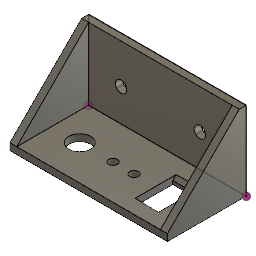
Switch Bracket v2 (Autodesk Fusion 360 design; units mm, degrees)
Autodesk Fusion 360 part; units mm, degrees
note: some values were not read from the file. Set by a fixed rule: which sketch regions a step uses.
sketch "Sketch1" plane through (0, 0, 0) normal (0, 1, 0) x (1, 0, 0)
  line L0 (45, 22.5) -> (-45, 22.5)
  line L1 (-45, 22.5) -> (-45, -22.5)
  line L2 (-45, -22.5) -> (45, -22.5)
  line L3 (45, -22.5) -> (45, 22.5)
  line L4 (45, 22.5) -> (-45, -22.5) construction
  line L5 (-45, 22.5) -> (45, -22.5) construction
  dimension "d1" = 45
  dimension "d2" = 90
  constraint perpendicular L0 L1
  constraint parallel L0 L2
  constraint parallel L1 L3
  constraint horizontal L0
  constraint coincident L4 origin
  constraint coincident L5 origin
  measures "d1" distance of L0.start L2.end L0.end
  measures "d2" distance of L0.start L0.end
extrude "Extrude1" add sketch "Sketch1" along normal blind 4
sketch "Sketch2" plane through (0, 0, -22.5) normal (0, 0, -1) x (-1, 0, 0)
  line L0 (45, 0) -> (-45, 0)
  line L1 (-45, 0) -> (-45, 45)
  line L2 (-45, 45) -> (45, 45)
  line L3 (45, 45) -> (45, 0)
  point P0 (-45, 0)
  point P1 (45, 0)
  dimension "d12" = 45
  constraint horizontal L0
  constraint vertical L1
  constraint horizontal L2
  constraint vertical L3
  constraint coincident L0 P0
  constraint coincident L1 P0
  constraint coincident L3 P1
  measures "d12" distance of P0 L1.end
extrude "Extrude4" add sketch "Sketch2" against normal blind 4
sketch "Sketch3" plane through (-45, 0, 0) normal (-1, 0, 0) x (0, 0, 1)
  line L0 (-22.5, 0) -> (22.5, 0)
  line L1 (22.5, 0) -> (22.5, 4)
  line L2 (22.5, 4) -> (-18.5, 4)
  line L3 (-22.5, 45) -> (-22.5, 0)
  line L4 (-18.5, 45) -> (-18.5, 4)
  line L5 (22.5, 4) -> (-18.5, 45)
  line L6 (-18.5, 4) -> (-18.5, 45)
  line L7 (-18.5, 45) -> (-22.5, 45)
  constraint coincident L2.end L4.end
  constraint coincident L1.end L2.start
  constraint coincident L4.start L5.end
extrude "Extrude3" add sketch "Sketch3" against normal blind 4 contours L2 L4 L5 L6
mirror "Mirror1" about plane through (0, 0, 0) normal (1, 0, 0) of "Extrude3"
sketch "Sketch4" plane through (0, 0, -18.5) normal (0, 0, 1) x (1, 0, 0)
  line L0 (41, 4) -> (41, 45)
  line L1 (41, 45) -> (-41, 45)
  line L2 (-41, 45) -> (-41, 4)
  line L3 (-41, 4) -> (41, 4)
  circle A0 centre (-22.5, 22.5) radius 3.25
  line L4 (-22.5, 22.5) -> (-16, 22.5) construction
  line L5 (45, 45) -> (-45, 45)
  line L6 (-45, 0) -> (45, 0)
  line L7 (0, 0) -> (0, 21) construction
  circle A1 centre (22.5, 22.5) radius 3.25
  dimension "d15" = 6.5
  dimension "d16" = 45
  constraint coincident A0.centre L4.start
  constraint horizontal L4
  constraint symmetric L4 L5 L6
  constraint coincident L7.start origin
  constraint perpendicular L3 L7
  constraint symmetric A0 L7 A1
  measures "d15" diameter of A0
  measures "d16" distance of A0.centre A1.centre
extrude "Extrude5" cut sketch "Sketch4" against normal through all contours A0 | A1
sketch "Sketch5" plane through (0, 0, 0) normal (0, -1, 0) x (1, 0, 0)
  line L0 (45, -22.5) -> (45, 22.5)
  line L1 (45, 22.5) -> (-45, 22.5)
  line L2 (-45, 22.5) -> (-45, -22.5)
  line L3 (-45, -22.5) -> (45, -22.5)
  circle A0 centre (-25, 2.5) radius 6.25
  line L4 (18.25, 12.25) -> (31.75, 12.25)
  line L5 (31.75, 12.25) -> (31.75, -7.25)
  line L6 (31.75, -7.25) -> (18.25, -7.25)
  line L7 (18.25, -7.25) -> (18.25, 12.25)
  line L8 (-25, 2.5) -> (31.5002, 2.5) construction
  line L9 (-45, -22.5) -> (45, -22.5)
  line L10 (25, -13) -> (25, 19) construction
  line L11 (-25, 2.5) -> (-25, -11) construction
  line L12 (0, 0) -> (0, -11) construction
  circle A1 centre (-6, 2.5) radius 2.5
  circle A2 centre (6, 2.5) radius 2.5
  dimension "d18" = 12.5
  dimension "d19" = 19.5
  dimension "d20" = 13.5
  dimension "d21" = 25
  dimension "d22" = 50
  dimension "d26" = 5
  dimension "d27" = 12
  constraint horizontal L4
  constraint vertical L5
  constraint horizontal L6
  constraint vertical L7
  constraint coincident A0.centre L8.start
  constraint horizontal L8
  constraint symmetric L4 L6 L8
  constraint perpendicular L4 L10
  constraint perpendicular L8 L11
  constraint coincident L12.start origin
  constraint vertical L12
  constraint coincident L8 A1.centre
  constraint symmetric L12 A1 A2
  measures "d18" diameter of A0
  measures "d19" distance of L4 L6
  measures "d20" distance of L4.start L4.end
  measures "d21" distance of L8 L9
  measures "d22" distance of A0.centre L10
  measures "d26" diameter of A1
  measures "d27" distance of A1.centre A2.centre
extrude "Extrude6" cut sketch "Sketch5" against normal blind 4 contours A0 | L4 L5 L6 L7 | A1 | A2
chamfer "Chamfer1" distance 2 angle 45 2 edges at (25, 4, -7.25) (25, 4, 12.25)
